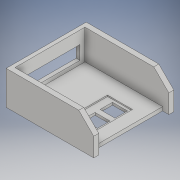
# Autodesk Inventor part: Base-Motherboard
Saved by Autodesk Inventor 2018 (Build 220112000, 112)
## iProperties
Created: 2017-07-20
Part Number: Base-Motherboard
Material: Generic
Document SubType Name: Modeling
Designer: JAck
Density: 1 g/cm^3
Appearance: Default
Author: JAck
Autodesk Inventor part; units mm, degrees
ref_plane "YZ Plane" through (0, 0, 0) normal (1, 0, 0) x (0, 1, 0)
ref_plane "XZ Plane" through (0, 0, 0) normal (0, 1, 0) x (-1, 0, 0)
ref_plane "XY Plane" through (0, 0, 0) normal (0, 0, 1) x (1, 0, 0)
sketch "Sketch1" plane through (0, 0, 0) normal (0, 1, 0) x (-1, 0, 0)
  line L0 (72.6415, 114.85) -> (-102.3585, 114.85)
  line L1 (-102.3585, 114.85) -> (-102.3585, -45.15)
  line L2 (-102.3585, -45.15) -> (72.6415, -45.15)
  line L3 (72.6415, -45.15) -> (72.6415, 114.85)
  line L4 (65.1415, 104.85) -> (-102.3585, 104.85)
  line L5 (-102.3585, 104.85) -> (-102.3585, -35.15)
  line L6 (-102.3585, -35.15) -> (65.1415, -35.15)
  line L7 (65.1415, -35.15) -> (65.1415, 104.85)
  line L8 (-102.3585, -35.15) -> (-89.8585, -35.15)
  line L9 (-89.8585, -35.15) -> (-89.8585, 104.85)
  line L10 (-89.8585, 104.85) -> (-102.3585, 104.85)
  line L11 (-102.3585, 104.85) -> (-102.3585, -35.15)
  point P0 (0, 0)
  dimension "d0" = 175
  dimension "d1" = 160
  dimension "d2" = 7.5
  dimension "d3" = 0
  dimension "d4" = 10
  dimension "d5" = 10
  dimension "d6" = 140
  dimension "d7" = 167.5
  dimension "d8" = 12.5
  constraints: 24 end point, 6 parallel, 3 horizontal, 3 perpendicular, 1 point on line
  measures "d0" distance between parallel lines of L1 L3
  measures "d1" distance of L0.end L1.end
  measures "d2" distance between parallel lines of L3 L7
  measures "d3" distance between parallel lines of L1 L5
  measures "d4" distance between parallel lines of L2 L6
  measures "d5" distance between parallel lines of L0 L4
  measures "d6" distance between parallel lines of L6 L4
  measures "d7" distance between parallel lines of L5 L7
  measures "d8" distance between parallel lines of L9 L1
extrude "Extrusion1" add sketch "Sketch1" along normal blind 60 contours L3 L2 L1 L6 L7 L4 L0
sketch "Sketch2" plane through (-72.6415, 0, -45.15) normal (-1, 0, 0) x (0, 0, 1)
  line L0 (20, 52.5) -> (140, 52.5)
  line L1 (140, 52.5) -> (140, 25)
  line L2 (140, 25) -> (20, 25)
  line L3 (20, 25) -> (20, 52.5)
  line L4 (160, 0) -> (160, 60) projected
  line L5 (0, 0) -> (0, 60) projected
  line L6 (0, 60) -> (160, 60) projected
  line L7 (0, 0) -> (160, 0) projected
  point P0 (45.15, 0)
  dimension "d11" = 20
  dimension "d12" = 20
  dimension "d13" = 7.5
  dimension "d14" = 25
  dimension "d15" = 120
  dimension "d16" = 27.5
  constraints: 8 end point, 2 parallel, 1 horizontal, 1 perpendicular
  measures "d11" distance between parallel lines of L4 L1
  measures "d12" distance between parallel lines of L5 L3
  measures "d13" distance between parallel lines of L6 L0
  measures "d14" distance between parallel lines of L7 L2
  measures "d15" distance between parallel lines of L3 L1
  measures "d16" distance of L0.end L1.end
extrude "Extrusion2" cut sketch "Sketch2" against normal blind 60 contours L0 L1 L2 L3
sketch "Sketch3" plane through (0, 60, 0) normal (0, 1, 0) x (1, 0, 0)
  line L0 (-72.6415, -114.85) -> (102.3585, -114.85) projected
  line L1 (102.3585, 45.15) -> (-72.6415, 45.15) projected
  line L2 (-72.6415, -114.85) -> (102.3585, -114.85)
  line L3 (102.3585, -114.85) -> (102.3585, 45.15)
  line L4 (102.3585, 45.15) -> (-72.6415, 45.15)
  line L5 (-72.6415, 45.15) -> (-72.6415, -114.85)
  point P0 (0, 0)
  constraints: 8 end point, 2 parallel, 1 horizontal, 1 perpendicular
extrude "Extrusion3" add sketch "Sketch3" along normal blind 7.5
sketch "Sketch4" plane through (0, 60, 0) normal (0, -1, 0) x (1, 0, 0)
  line L0 (-65.1415, 104.85) -> (102.3585, 104.85) projected
  line L1 (102.3585, -35.15) -> (-65.1415, -35.15) projected
  line L2 (102.3585, 104.85) -> (89.8585, 104.85)
  line L3 (89.8585, 104.85) -> (89.8585, -35.15)
  line L4 (89.8585, -35.15) -> (102.3585, -35.15)
  line L5 (102.3585, -35.15) -> (102.3585, 104.85)
  point P0 (0, 0)
  dimension "d21" = 12.5
  constraints: 8 end point, 2 parallel, 1 horizontal, 1 perpendicular, 1 point on line
  measures "d21" distance between parallel lines of L5 L3
extrude "Extrusion4" cut sketch "Sketch4" against normal blind 7.5
chamfer "Chamfer1" distance 30 angle 45 2 edges at (102.3585, 0, 109.85) (102.3585, 0, -40.15)
sketch "Sketch5" plane through (0, 67.5, 0) normal (0, 1, 0) x (1, 0, 0)
  line L0 (59.8585, -4.85) -> (29.8585, -4.85)
  line L1 (29.8585, -4.85) -> (29.8585, -29.85)
  line L2 (29.8585, -29.85) -> (59.8585, -29.85)
  line L3 (59.8585, -29.85) -> (59.8585, -4.85)
  line L4 (59.8585, -64.85) -> (29.8585, -64.85)
  line L5 (29.8585, -64.85) -> (29.8585, -39.85)
  line L6 (29.8585, -39.85) -> (59.8585, -39.85)
  line L7 (59.8585, -39.85) -> (59.8585, -64.85)
  line L8 (89.8585, -104.85) -> (89.8585, 35.15) projected
  line L9 (-72.6415, -114.85) -> (102.3585, -114.85) projected
  line L10 (102.3585, 45.15) -> (-72.6415, 45.15) projected
  point P0 (0, 0)
  dimension "d27" = 30
  dimension "d28" = 30
  dimension "d29" = 10
  dimension "d30" = 50
  dimension "d31" = 50
  dimension "d32" = 25
  dimension "d33" = 30
  dimension "d34" = 30
  constraints: 16 end point, 4 parallel, 2 horizontal, 2 perpendicular, 1 point on line
  measures "d27" distance between parallel lines of L8 L3
  measures "d28" distance between parallel lines of L8 L7
  measures "d29" distance between parallel lines of L6 L2
  measures "d30" distance between parallel lines of L9 L4
  measures "d31" distance between parallel lines of L10 L0
  measures "d32" distance of L0.end L1.end
  measures "d33" distance of L0.start L0.end
  measures "d34" distance between parallel lines of L7 L5
extrude "Extrusion5" cut sketch "Sketch5" against normal blind 7.5
sketch "Sketch6" plane through (0, 60, 0) normal (0, -1, 0) x (1, 0, 0)
  line L0 (64.8585, 69.85) -> (14.8585, 69.85)
  line L1 (14.8585, 69.85) -> (14.8585, -0.15)
  line L2 (14.8585, -0.15) -> (64.8585, -0.15)
  line L3 (64.8585, -0.15) -> (64.8585, 69.85)
  line L4 (59.8585, 64.85) -> (59.8585, 39.85) projected
  line L5 (29.8585, 39.85) -> (29.8585, 64.85) projected
  line L6 (29.8585, 64.85) -> (59.8585, 64.85) projected
  line L7 (59.8585, 4.85) -> (29.8585, 4.85) projected
  point P0 (0, 0)
  dimension "d37" = 5
  dimension "d38" = 15
  dimension "d39" = 5
  dimension "d40" = 5
  constraints: 8 end point, 2 parallel, 1 horizontal, 1 perpendicular
  measures "d37" distance between parallel lines of L3 L4
  measures "d38" distance between parallel lines of L5 L1
  measures "d39" distance between parallel lines of L6 L0
  measures "d40" distance between parallel lines of L2 L7
extrude "Extrusion6" cut sketch "Sketch6" against normal blind 2.5
equation "\"d5\" = d4"
equation "\"d12\" = d11"
equation "\"d30\" = d31"
equation "\"d34\" = d33"
body "Solid1"
